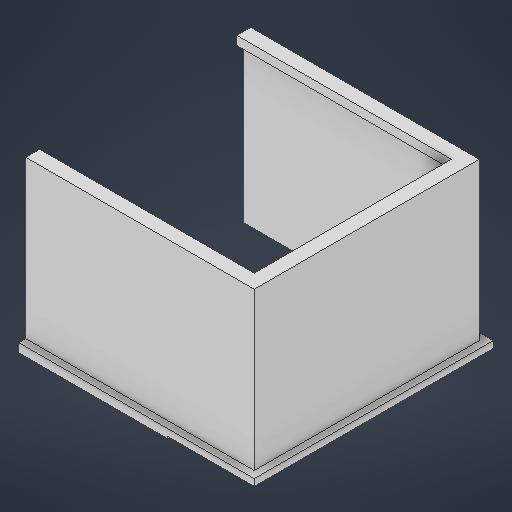
# Autodesk Inventor part: Galvo Housing-01
Saved by Autodesk Inventor 2025 (Build 290162000, 162)
## iProperties
Created: 2024-06-12
Part Number: Galvo Housing-01
Material: Generic
Document SubType Name: Modeling
Designer: mayhe
Density: 1 g/cm^3
Appearance: Default
Author: mayhe
Autodesk Inventor part; units mm, degrees
ref_plane "YZ Plane" through (0, 0, 0) normal (1, 0, 0) x (0, 1, 0)
ref_plane "XZ Plane" through (0, 0, 0) normal (0, 1, 0) x (-1, 0, 0)
ref_plane "XY Plane" through (0, 0, 0) normal (0, 0, 1) x (1, 0, 0)
sketch "Sketch8" plane through (0, 0, 0) normal (0, 1, 0) x (-1, 0, 0)
  line L0 (-65.5, -64.5) -> (65.5, -64.5)
  line L1 (65.5, -64.5) -> (65.5, 64.5)
  line L2 (65.5, 64.5) -> (-65.5, 64.5)
  line L3 (-65.5, 64.5) -> (-65.5, -64.5)
  line L4 (-65.5, -64.5) -> (65.5, 64.5) construction
  line L5 (65.5, -64.5) -> (-65.5, 64.5) construction
  point P0 (0, 0)
  dimension "d26" = 131
  dimension "d27" = 129
  constraints: 12 end point, 2 midpoint, 2 parallel, 1 horizontal, 1 perpendicular
  measures "d26" distance of L2.end L1.end
  measures "d27" distance of L1.end L0.end
extrude "Extrusion7" add sketch "Sketch8" along normal blind 95
sketch "Sketch9" plane through (0, 0, 0) normal (0, -1, 0) x (1, 0, 0)
  line L0 (-65.5, 64.5) -> (65.5, 64.5) projected
  line L1 (-65.5, -64.5) -> (65.5, -64.5)
  line L2 (65.5, -64.5) -> (65.5, 64.5)
  line L3 (65.5, 64.5) -> (-65.5, 64.5)
  line L4 (-65.5, 64.5) -> (-65.5, -64.5)
  line L5 (-65.5, -64.5) -> (65.5, 64.5) construction
  line L6 (65.5, -64.5) -> (-65.5, 64.5) construction
  line L7 (61.5, 60.5) -> (61.5, -60.5)
  line L8 (61.5, -60.5) -> (-65.5, -60.5)
  line L9 (-65.5, 60.5) -> (61.5, 60.5)
  line L10 (57.5, -56.5) -> (57.5, 56.5)
  line L11 (57.5, 56.5) -> (-65.5, 56.5)
  line L12 (-65.5, -56.5) -> (57.5, -56.5)
  line L13 (-63.4537, -60.5) -> (-63.4537, -62.485)
  line L14 (-63.4537, 62.485) -> (-63.4537, 60.5)
  line L15 (-59.3922, 56.5) -> (-59.3922, 58.4854)
  line L16 (-59.3922, -58.4854) -> (-59.3922, -56.5)
  point P0 (0, 0)
  dimension "d30" = 4
  dimension "d31" = 4
  dimension "d47" = 4
  dimension "d48" = 4
  dimension "d49" = 4
  dimension "d50" = 4
  constraints: 32 end point, 12 point on line, 8 parallel, 3 perpendicular, 2 midpoint, 1 horizontal
  measures "d30" distance between parallel lines of L2 L7
  measures "d31" distance between parallel lines of L7 L10
  measures "d47" distance between parallel lines of L0 L9
  measures "d48" distance between parallel lines of L11 L9
  measures "d49" distance between parallel lines of L1 L8
  measures "d50" distance between parallel lines of L8 L12
extrude "Extrusion8" cut sketch "Sketch9" against normal blind 115 contours L11 L10 L12 L4
extrude "Extrusion9" cut sketch "Sketch9" against normal blind 90 contours L9 L7 L8 L4 L12 L10 L11
sketch "Sketch10" plane through (0, 0, 0) normal (0, -1, 0) x (1, 0, 0)
  line L0 (65.5, -64.5) -> (-65.5, -64.5)
  line L1 (-65.5, -64.5) -> (-65.5, 64.5)
  line L2 (-65.5, 64.5) -> (65.5, 64.5)
  line L3 (65.5, 64.5) -> (65.5, -64.5)
  line L4 (65.5, -64.5) -> (-65.5, 64.5) construction
  line L5 (-65.5, -64.5) -> (65.5, 64.5) construction
  line L6 (-69.5, 68.5) -> (-69.5, -68.5)
  line L7 (-69.5, -68.5) -> (69.5, -68.5)
  line L8 (69.5, -68.5) -> (69.5, 68.5)
  line L9 (69.5, 68.5) -> (-69.5, 68.5)
  line L10 (-65.5, 64.5) -> (-69.5, 64.5)
  line L11 (-65.5, -64.5) -> (-69.5, -64.5)
  line L12 (-65.5, 64.5) -> (-65.5, 68.5)
  line L13 (-65.5, -64.5) -> (-65.5, -68.5)
  point P0 (0, 0)
  dimension "d36" = 4
  constraints: 28 end point, 5 perpendicular, 5 point on line, 4 parallel, 2 midpoint, 1 horizontal, 3 other
  measures "d36" distance between parallel lines of L1 L6
extrude "Extrusion10" add sketch "Sketch10" against normal blind 5 contours L3 L2 L12 L9 L8 L7 L13 L0
sketch "Sketch11" plane through (0, 0, 0) normal (0, -1, 0) x (1, 0, 0)
  circle A0 centre (-66.5, 0.5) radius 135
  line L0 (61.5, 60.5) -> (61.5, -60.5) projected
  line L1 (69.5, -68.5) -> (69.5, 68.5) projected
  circle A1 centre (-66.5, 0.5) radius 110
  line L2 (19.168, -68.5) -> (69.5, -68.5)
  line L3 (69.5, -68.5) -> (69.5, 68.5)
  line L4 (69.5, 68.5) -> (19.9639, 68.5)
  line L5 (-65.5, 68.5) -> (69.5, 68.5) projected
  point P0 (0, 0)
  dimension "d39" = 270
  dimension "d41" = 136
  dimension "d42" = 220
  constraints: 6 end point, 2 centre point, 2 point on circle, 1 coincident, 1 collinear, 1 perpendicular, 1 point on line
  measures "d39" diameter of A0
  measures "d41" distance from line of L1 A0.centre
  measures "d42" diameter of A1
extrude "Extrusion11" cut sketch "Sketch11" against normal blind 1.125 contours A0 L0 | A0 L4 L1 L2 | L0 A0 L2 A1 L4
body "Solid3"
